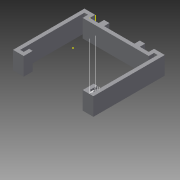
# Autodesk Inventor part: Up go er
Saved by Autodesk Inventor 2015 (Build 190159000, 159)
## iProperties
Created: 2016-05-27
Part Number: Up go er
Material: Generic
Document SubType Name: Modeling
Designer: Toby
Density: 1 g/cm^3
Appearance: Default
Author: Toby
Autodesk Inventor part; units mm, degrees
ref_plane "YZ Plane" through (0, 0, 0) normal (1, 0, 0) x (0, 1, 0)
ref_plane "XZ Plane" through (0, 0, 0) normal (0, 1, 0) x (-1, 0, 0)
ref_plane "XY Plane" through (0, 0, 0) normal (0, 0, 1) x (1, 0, 0)
sketch "Sketch1" plane through (0, 0, 0) normal (0, 0, 1) x (1, 0, 0)
  line L0 (-23.4921, 12.3401) -> (-21.4921, 12.3401)
  line L1 (-21.4921, 12.3401) -> (-21.4921, -27.6599)
  line L2 (-21.4921, -27.6599) -> (-23.4921, -27.6599)
  line L3 (-23.4921, -27.6599) -> (-23.4921, 12.3401)
  line L4 (-23.4921, -27.6599) -> (-17.4921, -27.6599)
  line L5 (-17.4921, -27.6599) -> (-17.4921, -25.6599)
  line L6 (-17.4921, -25.6599) -> (-23.4921, -25.6599)
  line L7 (-23.4921, -25.6599) -> (-23.4921, -27.6599)
  line L8 (-17.4921, -27.6599) -> (-19.4921, -27.6599)
  line L9 (-19.4921, -27.6599) -> (-19.4921, -22.6599)
  line L10 (-19.4921, -22.6599) -> (-17.4921, -22.6599)
  line L11 (-17.4921, -22.6599) -> (-17.4921, -27.6599)
  line L12 (-23.4921, 12.3401) -> (-17.4921, 12.3401)
  line L13 (-17.4921, 12.3401) -> (-17.4921, 10.3401)
  line L14 (-17.4921, 10.3401) -> (-23.4921, 10.3401)
  line L15 (-23.4921, 10.3401) -> (-23.4921, 12.3401)
  line L16 (-17.4921, 12.3401) -> (-19.4921, 12.3401)
  line L17 (-19.4921, 12.3401) -> (-19.4921, 7.3401)
  line L18 (-19.4921, 7.3401) -> (-17.4921, 7.3401)
  line L19 (-17.4921, 7.3401) -> (-17.4921, 12.3401)
  line L20 (-19.4921, 9.3401) -> (17.5079, 9.3401)
  line L21 (17.5079, 9.3401) -> (17.5079, 7.3401)
  line L22 (17.5079, 7.3401) -> (-19.4921, 7.3401)
  line L23 (-19.4921, 7.3401) -> (-19.4921, 9.3401)
  line L24 (17.5079, 7.3401) -> (15.5079, 7.3401)
  line L25 (15.5079, 7.3401) -> (15.5079, 12.3401)
  line L26 (15.5079, 12.3401) -> (17.5079, 12.3401)
  line L27 (17.5079, 12.3401) -> (17.5079, 7.3401)
  line L28 (15.5079, 12.3401) -> (21.5079, 12.3401)
  line L29 (21.5079, 12.3401) -> (21.5079, 10.3401)
  line L30 (21.5079, 10.3401) -> (15.5079, 10.3401)
  line L31 (15.5079, 10.3401) -> (15.5079, 12.3401)
  line L32 (21.5079, 12.3401) -> (19.5079, 12.3401)
  line L33 (19.5079, 12.3401) -> (19.5079, -27.6599)
  line L34 (19.5079, -27.6599) -> (21.5079, -27.6599)
  line L35 (21.5079, -27.6599) -> (21.5079, 12.3401)
  line L36 (21.5079, -27.6599) -> (15.5079, -27.6599)
  line L37 (15.5079, -27.6599) -> (15.5079, -25.7551)
  line L38 (15.5079, -25.7551) -> (21.5079, -25.7551)
  line L39 (21.5079, -25.7551) -> (21.5079, -27.6599)
  line L40 (15.5079, -27.6599) -> (17.5079, -27.6599)
  line L41 (17.5079, -27.6599) -> (17.5079, -21.4921)
  line L42 (17.5079, -21.4921) -> (15.5079, -21.4921)
  line L43 (15.5079, -21.4921) -> (15.5079, -27.6599)
  point P0 (0, 0)
  dimension "d0" = 40
  dimension "d1" = 2
  dimension "d2" = 2
  dimension "d3" = 2
  dimension "d4" = 2
  dimension "d5" = 5
  dimension "d6" = 5
  dimension "d7" = 37
  dimension "d8" = 6
  dimension "d9" = 6
  dimension "d10" = 2
  dimension "d11" = 2
  dimension "d12" = 2
  dimension "d13" = 2
  dimension "d14" = 2
  dimension "d15" = 40
  dimension "d16" = 6
  dimension "d17" = 6
  dimension "d18" = 45
  constraints: 88 end point, 22 parallel, 11 horizontal, 11 perpendicular, 4 point on line
  measures "d0" distance of L2.end L0.start
  measures "d1" distance between parallel lines of L3 L1
  measures "d2" distance between parallel lines of L35 L33
  measures "d3" distance between parallel lines of L12 L14
  measures "d4" distance between parallel lines of L4 L6
  measures "d5" distance of L8.end L9.end
  measures "d6" distance of L16.end L17.end
  measures "d7" distance of L21.end L22.end
  measures "d8" distance of L0.start L12.end
  measures "d9" distance of L25.end L28.end
  measures "d10" distance from line of L27 L30.end
  measures "d11" distance between parallel lines of L19 L17
  measures "d12" distance between parallel lines of L22 L20
  measures "d13" distance between parallel lines of L11 L9
  measures "d14" distance between parallel lines of L43 L41
  measures "d15" distance of L32.end L33.end
  measures "d16" distance of L5.end L6.end
  measures "d17" distance of L37.end L38.end
  measures "d18" distance between parallel lines of L35 L3
extrude "Extrusion1" add sketch "Sketch1" along normal blind 10
sketch "Sketch2" plane through (-17.4921, 9.3401, 0) normal (1, 0, 0) x (0, 0, -1)
  line L0 (-10, 0) -> (0, 0) projected
  line L1 (0, 3) -> (-10, 3) projected
  point P0 (0, -9.3401)
  dimension "d21" = 3
  measures "d21" distance between parallel lines of L0 L1
sketch "Sketch3" plane through (-17.4921, 9.3401, 0) normal (0, 1, 0) x (1, 0, 0)
  line L0 (-2, -10) -> (35, -10) projected
  line L1 (5, 0) -> (8, 0)
  line L2 (8, 0) -> (8, -10)
  line L3 (8, -10) -> (5, -10)
  line L4 (5, -10) -> (5, 0)
  line L5 (28, 0) -> (25, 0)
  line L6 (25, 0) -> (25, -10)
  line L7 (25, -10) -> (28, -10)
  line L8 (28, -10) -> (28, 0)
  line L9 (0, 0) -> (0, -10) projected
  line L10 (33, 0) -> (33, -10) projected
  point P0 (17.4921, 0)
  dimension "d22" = 5
  dimension "d23" = 5
  dimension "d24" = 3
  dimension "d25" = 3
  constraints: 16 end point, 4 parallel, 3 point on line, 2 horizontal, 2 perpendicular
  measures "d22" distance between parallel lines of L9 L4
  measures "d23" distance between parallel lines of L10 L8
  measures "d24" distance of L5.start L5.end
  measures "d25" distance of L1.start L1.end
extrude "Extrusion2" add sketch "Sketch3" along normal blind 3
body "Solid1"
